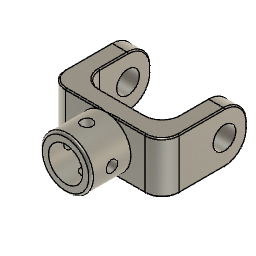
bracket v2 (Autodesk Fusion 360 design; units mm, degrees)
Autodesk Fusion 360 part; units mm, degrees
sketch "Sketch2" plane through (0, 0, 0) normal (0, 0, 1) x (1, 0, 0)
  line L0 (0, 0) -> (100, 0)
  line L1 (100, 0) -> (100, 150)
  line L2 (100, 150) -> (70, 150)
  line L3 (70, 150) -> (70, 30)
  line L4 (70, 30) -> (0, 30)
  line L5 (0, 2.5) -> (0, 20)
  line L6 (-100, 150) -> (-70, 150)
  line L7 (-70, 30) -> (0, 30)
  line L8 (0, 0) -> (-100, 0)
  line L9 (-100, 0) -> (-100, 150)
  line L10 (-70, 150) -> (-70, 30)
  dimension "d15" = 100
  dimension "d16" = 150
  dimension "d17" = 30
  dimension "d18" = 120
  dimension "d19" = 70
  constraint coincident L0.start L8.start
  constraint horizontal L0
  constraint perpendicular L0 L1
  constraint perpendicular L1 L2
  constraint perpendicular L2 L3
  constraint perpendicular L3 L4
  constraint symmetric L0.start L5 L8.start
  constraint symmetric L0.end L5 L8.end
  constraint symmetric L1.end L5 L6.start
  constraint symmetric L2.end L5 L6.end
  constraint symmetric L3.end L5 L7.start
  constraint symmetric L4.end L5 L7.end
  measures "d15" distance of L0.start L0.end
  measures "d16" distance of L0.end L1.end
  measures "d17" distance of L1.end L2.end
  measures "d18" distance of L2.end L3.end
  measures "d19" distance of L3.end L4.end
extrude "Extrude3" add sketch "Sketch2" along normal blind 90
fillet "Fillet2" radius 40 1 edges at (85, 150, 90)
fillet "Fillet3" radius 40 1 edges at (85, 150, 0)
fillet "Fillet4" radius 40 1 edges at (-85, 150, 90)
fillet "Fillet5" radius 40 1 edges at (-85, 150, 0)
sketch "Sketch3" plane through (0, 0, 0) normal (0, -1, 0) x (1, 0, 0)
  line L0 (-100, 0) -> (100, 0)
  line L1 (100, 0) -> (100, 90)
  line L2 (100, 90) -> (-100, 90)
  line L3 (-100, 90) -> (-100, 0)
  circle A0 centre (0, 45) radius 45
  dimension "d30" = 90
  constraint tangent L2 A0
  constraint vertical origin A0.centre
  measures "d30" diameter of A0
extrude "Extrude4" add sketch "Sketch3" along normal blind 70 contours A0
fillet "Fillet6" radius 4 1 edges at (-41.9547, -70, 28.7273)
fillet "Fillet7" radius 30 1 edges at (100, 0, 45)
fillet "Fillet8" radius 30 3 edges at (-100, 0, 45) (-70, 30, 45) (70, 30, 45)
sketch "Sketch4" plane through (0, -70, 0) normal (0, -1, 0) x (1, 0, 0)
  circle A0 centre (0, 45) radius 41
  circle A1 centre (0, 45) radius 30
  dimension "d39" = 60
  constraint concentric A0 A1
  measures "d39" diameter of A1
extrude "Extrude5" cut sketch "Sketch4" against normal blind 100 contours A1
sketch "Sketch5" plane through (0, 0, 0) normal (0, 0, 1) x (1, 0, 0)
  circle A0 centre (0, -33) radius 10
  dimension "d43" = 33
  dimension "d44" = 20
  measures "d43" distance of origin A0.centre
  measures "d44" diameter of A0
extrude "Extrude6" cut sketch "Sketch5" along normal through all
pattern_circular "C-Pattern1" count 4 over 360 about axis through (0, -70, 45) along (0, 1, 0) of "Extrude6"
sketch "Sketch6" plane through (100, 0, 0) normal (1, 0, 0) x (0, 1, 0)
  line L0 (30, 90) -> (30, 0)
  line L1 (30, 0) -> (110, 0)
  arc A0 (110, 0) -> (150, 40) centre (110, 40) ccw
  line L2 (150, 40) -> (150, 50)
  arc A1 (150, 50) -> (110, 90) centre (110, 50) ccw
  line L3 (110, 90) -> (30, 90)
  circle A2 centre (110, 45) radius 20
  dimension "d50" = 45
  dimension "d51" = 40
  measures "d50" distance of A1.end A2.centre
  measures "d51" diameter of A2
extrude "Extrude7" cut sketch "Sketch6" against normal through all contours A2
fillet "Fillet9" radius 2 18 edges at (35, 0, 90) (91.2132, 8.7868, 90) (100, 70, 90) (100, 138.2843, 78.2843) (100, 150, 45) (100, 138.2843, 11.7157) (100, 70, 0) (91.2132, 8.7868, 0) (35, 0, 0) (-35, 0, 0) (-91.2132, 8.7868, 0) (-100, 70, 0) (-100, 138.2843, 11.7157) (-100, 150, 45) (-100, 138.2843, 78.2843) (-100, 70, 90) (-91.2132, 8.7868, 90) (-35, 0, 90)
fillet "Fillet10" radius 2 16 edges at (-61.2132, 38.7868, 90) (-70, 85, 90) (-70, 138.2843, 78.2843) (-70, 150, 45) (-70, 138.2843, 11.7157) (-70, 85, 0) (-61.2132, 38.7868, 0) (0, 30, 0) (61.2132, 38.7868, 0) (70, 85, 0) (70, 138.2843, 11.7157) (70, 150, 45) (70, 138.2843, 78.2843) (70, 85, 90) (61.2132, 38.7868, 90) (0, 30, 90)
